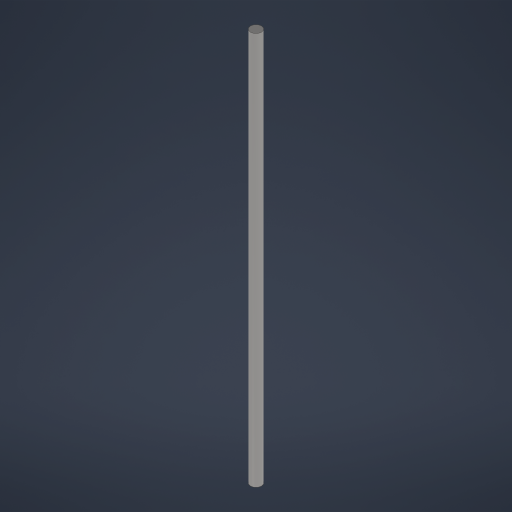
# Autodesk Inventor part: bar
Saved by Autodesk Inventor 2023 (Build 270158000, 158)
## iProperties
Created: 2022-04-23
Part Number: bar
Material: Stainless Steel
Document SubType Name: Modeling
Designer: Norbert Ligas
Density: 8 g/cm^3
Appearance: Semi-Polished
bar_length: 285,000
bar_diameter: 8,000 mm
Author: Norbert Ligas
Autodesk Inventor part; units mm, degrees
ref_plane "YZ Plane" through (0, 0, 0) normal (1, 0, 0) x (0, 1, 0)
ref_plane "XZ Plane" through (0, 0, 0) normal (0, 1, 0) x (-1, 0, 0)
ref_plane "XY Plane" through (0, 0, 0) normal (0, 0, 1) x (1, 0, 0)
sketch "Sketch1" plane through (0, 0, 0) normal (0, 1, 0) x (-1, 0, 0)
  circle A0 centre (0, 0) radius 4
  dimension "d0" = 8
  constraints: 1 centre point, 1 coincident
  measures "d0" diameter of A0
extrude "Extrusion1" add sketch "Sketch1" along normal blind 285
equation "\"d0\" = bar_diameter"
equation "\"d1\" = bar_length"
equation "\"bar_length\" = 285"
equation "\"bar_diameter\" = 8"
body "Solid1"
